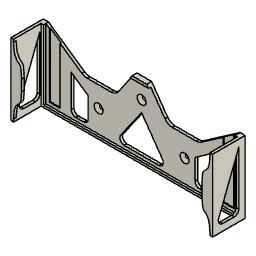
ThinkPad_Dock_Mount_v1 (Autodesk Fusion 360 design; units mm, degrees)
Autodesk Fusion 360 part; units mm, degrees
sketch "Sketch2" plane through (0, 0, 0) normal (0, 0, 1) x (1, 0, 0)
  line L0 (-139.5, 128) -> (87, 128)
  line L1 (87, 128) -> (87, 91.5)
  line L2 (87, 91.5) -> (-139.5, 91.5)
  line L3 (-139.5, 91.5) -> (-139.5, 128)
  line L4 (-136.5, 125) -> (84, 125)
  line L5 (84, 125) -> (84, 94.5)
  line L6 (84, 94.5) -> (-136.5, 94.5)
  line L7 (-136.5, 94.5) -> (-136.5, 125)
  dimension "d3" = 3
  dimension "d4" = 3
  dimension "d5" = 3
  dimension "d6" = 3
  dimension "d7" = 220.5
  dimension "d8" = 30.5
  constraint horizontal L0
  constraint vertical L1
  constraint horizontal L2
  constraint vertical L3
  constraint horizontal L4
  constraint vertical L5
  constraint horizontal L6
  constraint vertical L7
  measures "d3" distance of L0 L4
  measures "d4" distance of L1 L5
  measures "d5" distance of L3 L7
  measures "d6" distance of L2 L6
  measures "d7" distance of L5 L7
  measures "d8" distance of L4 L6
extrude "Extrude1" add sketch "Sketch2" along normal blind 80.5 makes body 1
sketch "Sketch3" plane through (0, 0, 0) normal (0, 0, -1) x (1, 0, 0)
  line L0 (-136.5, -94.5) -> (84, -94.5)
  line L1 (84, -94.5) -> (84, -125)
  line L2 (84, -125) -> (-136.5, -125)
  line L3 (-136.5, -125) -> (-136.5, -94.5)
  line L4 (87, -91.5) -> (-139.5, -91.5)
  line L5 (-139.5, -91.5) -> (-139.5, -128)
  line L6 (-139.5, -128) -> (87, -128)
  line L7 (87, -128) -> (87, -91.5)
  line L8 (-136.5, -125) -> (-133.75, -125)
  line L9 (-133.75, -125) -> (-133.75, -122.5)
  line L10 (-133.75, -122.5) -> (-136.5, -122.5)
  line L11 (-136.5, -122.5) -> (-136.5, -125)
  line L12 (84, -125) -> (81.25, -125)
  line L13 (81.25, -125) -> (81.25, -122.5)
  line L14 (81.25, -122.5) -> (84, -122.5)
  line L15 (84, -122.5) -> (84, -125)
  dimension "d11" = 2.5
  dimension "d12" = 2.75
  dimension "d13" = 2.5
  dimension "d14" = 2.75
  constraint horizontal L8
  constraint vertical L9
  constraint horizontal L10
  constraint vertical L11
  constraint coincident L2.end L3.start
  constraint horizontal L12
  constraint vertical L13
  constraint horizontal L14
  constraint vertical L15
  constraint coincident L1.end L2.start
  measures "d11" distance of L8 L10
  measures "d12" distance of L9 L11
  measures "d13" distance of L12 L14
  measures "d14" distance of L13 L15
extrude "Extrude2" add sketch "Sketch3" against normal blind 80.5 separate body contours L2 L3 L8 L9 L10 L11 | L1 L2 L12 L13 L14 L15 makes body 2 at (-134.6667, 122.5, 53.6667) makes body 3 at (83.0833, 125, 53.6667)
sketch "Sketch4" plane through (-133.75, 0, 0) normal (1, 0, 0) x (0, 1, 0)
  line L0 (122.5, 0) -> (125, 0)
  line L1 (125, 0) -> (125, 80.5)
  line L2 (125, 80.5) -> (122.5, 80.5)
  line L3 (122.5, 80.5) -> (122.5, 0)
  line L4 (122.5, 0) -> (125, 0)
  line L5 (125, 0) -> (125, 2.5)
  line L6 (125, 2.5) -> (122.5, 2.5)
  line L7 (122.5, 2.5) -> (122.5, 0)
  dimension "d17" = 2.5
  constraint horizontal L4
  constraint vertical L5
  constraint horizontal L6
  constraint vertical L7
  constraint coincident L1 L5.end
  constraint coincident L0.start L3.end
  measures "d17" distance of L4 L6
extrude "Extrude3" add sketch "Sketch4" along normal up to surface (215 mm away) contours L0 L1 L3 L4 L5 L6 L7 bodies 1 2 3
sketch "Sketch34" plane through (0, 91.5, 0) normal (0, -1, 0) x (1, 0, 0)
  line L0 (-139.5, 0) -> (87, 0)
  line L1 (-139.5, 80.5) -> (-139.5, 0)
  line L2 (-136.5, 2.753) -> (-136.5, 0)
  line L3 (-139.5, 40.25) -> (-127.5, 40.25)
  line L4 (-26.25, 0) -> (-26.25, 10)
  line L5 (-127.5, 40.25) -> (-127.5, 34.253)
  spline S0 degree 5 poles (-127.5, 34.253) (-127.5, 33.9218) (-127.5144, 33.2317) (-127.5794, 32.1133) (-127.7268, 30.4836) (-127.9198, 28.3513) (-128.0379, 26.2907) (-128.1709, 24.3948) (-128.4617, 22.7323) (-129.6807, 21.0236) (-131.358, 19.6123) (-132.5708, 18.9131) (-132.5285, 19.155) (-132.375, 19.0496) (-133.1587, 17.6828) (-134.3735, 15.6105) (-135.3998, 13.5294) (-135.6827, 12.0317) (-135.798, 10.5363) (-135.9647, 8.8274) (-136.2123, 6.8844) (-136.4008, 5.2251) (-136.482, 3.9805) (-136.5, 3.1606) (-136.5, 2.753) knots 0 0 0 0 0 0 0.05 0.1 0.15 0.2 0.25 0.3 0.35 0.4 0.45 0.5 0.55 0.6 0.65 0.7 0.75 0.8 0.85 0.9 0.95 1 1 1 1 1 1
  line L6 (-127.5, 37.2515) -> (-127.5, 31.2546)
  line L7 (-136.5, 6.6399) -> (-136.5, -1.1338)
  line L8 (-127.3272, 26.6249) -> (-129.6728, 19.7501)
  line L9 (-132.4893, 19.089) -> (-132.5107, 19.0556)
  line L10 (-134.7118, 16.064) -> (-136.2882, 9.4421)
  line L11 (-136.5, 77.747) -> (-136.5, 80.5)
  spline S1 degree 5 poles (-127.5, 46.247) (-127.5, 46.5782) (-127.5144, 47.2683) (-127.5794, 48.3867) (-127.7268, 50.0164) (-127.9198, 52.1487) (-128.0379, 54.2093) (-128.1709, 56.1052) (-128.4617, 57.7677) (-129.6807, 59.4764) (-131.358, 60.8877) (-132.5708, 61.5869) (-132.5285, 61.345) (-132.375, 61.4504) (-133.1587, 62.8172) (-134.3735, 64.8895) (-135.3998, 66.9706) (-135.6827, 68.4683) (-135.798, 69.9637) (-135.9647, 71.6726) (-136.2123, 73.6156) (-136.4008, 75.2749) (-136.482, 76.5195) (-136.5, 77.3394) (-136.5, 77.747) knots 0 0 0 0 0 0 0.05 0.1 0.15 0.2 0.25 0.3 0.35 0.4 0.45 0.5 0.55 0.6 0.65 0.7 0.75 0.8 0.85 0.9 0.95 1 1 1 1 1 1
  line L12 (-127.5, 43.2485) -> (-127.5, 49.2454)
  line L13 (-127.3272, 53.8751) -> (-129.6728, 60.7499)
  line L14 (-132.4893, 61.411) -> (-132.5107, 61.4444)
  line L15 (-134.7118, 64.436) -> (-136.2882, 71.0579)
  line L16 (-136.5, 73.8601) -> (-136.5, 81.6338)
  line L17 (-127.5, 40.25) -> (-127.5, 46.247)
  line L18 (84, 2.753) -> (84, 0)
  spline S2 degree 5 poles (75, 34.253) (75, 33.9218) (75.0144, 33.2317) (75.0794, 32.1133) (75.2268, 30.4836) (75.4198, 28.3513) (75.5379, 26.2907) (75.6709, 24.3948) (75.9617, 22.7323) (77.1807, 21.0236) (78.858, 19.6123) (80.0708, 18.9131) (80.0285, 19.155) (79.875, 19.0496) (80.6587, 17.6828) (81.8735, 15.6105) (82.8998, 13.5294) (83.1827, 12.0317) (83.298, 10.5363) (83.4647, 8.8274) (83.7123, 6.8844) (83.9008, 5.2251) (83.982, 3.9805) (84, 3.1606) (84, 2.753) knots 0 0 0 0 0 0 0.05 0.1 0.15 0.2 0.25 0.3 0.35 0.4 0.45 0.5 0.55 0.6 0.65 0.7 0.75 0.8 0.85 0.9 0.95 1 1 1 1 1 1
  line L19 (75, 37.2515) -> (75, 31.2546)
  line L20 (74.8272, 26.6249) -> (77.1728, 19.7501)
  line L21 (79.9893, 19.089) -> (80.0107, 19.0556)
  line L22 (82.2118, 16.064) -> (83.7882, 9.4421)
  line L23 (84, 6.6399) -> (84, -1.1338)
  line L24 (75, 40.25) -> (75, 34.253)
  line L25 (75, 40.25) -> (75, 46.247)
  spline S3 degree 5 poles (75, 46.247) (75, 46.5782) (75.0144, 47.2683) (75.0794, 48.3867) (75.2268, 50.0164) (75.4198, 52.1487) (75.5379, 54.2093) (75.6709, 56.1052) (75.9617, 57.7677) (77.1807, 59.4764) (78.858, 60.8877) (80.0708, 61.5869) (80.0285, 61.345) (79.875, 61.4504) (80.6587, 62.8172) (81.8735, 64.8895) (82.8998, 66.9706) (83.1827, 68.4683) (83.298, 69.9637) (83.4647, 71.6726) (83.7123, 73.6156) (83.9008, 75.2749) (83.982, 76.5195) (84, 77.3394) (84, 77.747) knots 0 0 0 0 0 0 0.05 0.1 0.15 0.2 0.25 0.3 0.35 0.4 0.45 0.5 0.55 0.6 0.65 0.7 0.75 0.8 0.85 0.9 0.95 1 1 1 1 1 1
  line L26 (75, 43.2485) -> (75, 49.2454)
  line L27 (74.8272, 53.8751) -> (77.1728, 60.7499)
  line L28 (79.9893, 61.411) -> (80.0107, 61.4444)
  line L29 (82.2118, 64.436) -> (83.7882, 71.0579)
  line L30 (84, 73.8601) -> (84, 81.6338)
  line L31 (84, 77.747) -> (84, 80.5)
  line L32 (-139.5, 80.5) -> (87, 80.5)
  point P0 (-127.5, 34.253)
  point P1 (-128.5, 23.1875)
  point P2 (-132.5, 19.0723)
  point P3 (-135.5, 12.753)
  point P4 (-136.5, 2.753)
  point P5 (-128.5, 23.1875)
  point P6 (-132.5, 19.0723)
  point P7 (-135.5, 12.753)
  point P8 (-128.5, 57.3125)
  point P9 (-132.5, 61.4277)
  point P10 (-135.5, 67.747)
  point P11 (76, 23.1875)
  point P12 (80, 19.0723)
  point P13 (83, 12.753)
  point P14 (76, 57.3125)
  point P15 (80, 61.4277)
  point P16 (83, 67.747)
  dimension "d201" = 3
  dimension "d255" = 12
  dimension "d257" = 11
  dimension "d259" = 7
  dimension "d261" = 4
  dimension "d263" = 3
  dimension "d265" = 3
  dimension "d266" = 18.839
  dimension "d267" = 32.677
  dimension "d268" = 13.391
  dimension "d274" = 41.3838
  constraint coincident L0 L2.end
  constraint midpoint L1 L3.start
  constraint perpendicular L1 L3
  constraint midpoint L0 L4.start
  constraint perpendicular L0 L4
  constraint coincident P0 L5.end
  constraint perpendicular L3 L5
  constraint coincident P5 P1
  constraint coincident P6 P2
  constraint coincident P7 P3
  constraint midpoint P0 L6
  constraint midpoint L5 L6.start
  constraint midpoint L2.start L7
  constraint midpoint P5 L8
  constraint midpoint P6 L9
  constraint midpoint P7 L10
  constraint parallel L1 L7
  constraint symmetric L2.start L3 L11.start
  constraint symmetric L2.end L3 L11.end
  constraint symmetric L5.start L3 L17.start
  constraint symmetric L3 P0 S1.start
  constraint symmetric L3 P5 P8
  constraint symmetric L3 P6 P9
  constraint symmetric L3 P7 P10
  constraint symmetric L3 L6.start L12.start
  constraint symmetric L3 L6.end L12.end
  constraint symmetric L3 L7.start L16.start
  constraint symmetric L3 L7.end L16.end
  constraint symmetric L3 L8.start L13.start
  constraint symmetric L3 L8.end L13.end
  constraint symmetric L3 L9.start L14.start
  constraint symmetric L3 L9.end L14.end
  constraint symmetric L3 L10.start L15.start
  constraint symmetric L3 L10.end L15.end
  constraint symmetric L2.start L4 L18.start
  constraint symmetric L2.end L4 L18.end
  constraint symmetric L3.end L4 L24.start
  constraint symmetric L4 P0 S2.start
  constraint symmetric L4 P5 P11
  constraint symmetric L4 P6 P12
  constraint symmetric L4 P7 P13
  constraint symmetric L4 L6.start L19.start
  constraint symmetric L4 L6.end L19.end
  constraint symmetric L4 L7.start L23.start
  constraint symmetric L4 L7.end L23.end
  constraint symmetric L4 L8.start L20.start
  constraint symmetric L4 L8.end L20.end
  constraint symmetric L4 L9.start L21.start
  constraint symmetric L4 L9.end L21.end
  constraint symmetric L4 L10.start L22.start
  constraint symmetric L4 L10.end L22.end
  constraint symmetric L4 L11.start S3.end
  constraint symmetric L4 L11.end L31.end
  constraint symmetric L4 S1.start L25.end
  constraint symmetric L4 P8 P14
  constraint symmetric L4 P9 P15
  constraint symmetric L4 P10 P16
  constraint symmetric L4 L12.start L26.start
  constraint symmetric L4 L12.end L26.end
  constraint symmetric L4 L13.start L27.start
  constraint symmetric L4 L13.end L27.end
  constraint symmetric L4 L14.start L28.start
  constraint symmetric L4 L14.end L28.end
  constraint symmetric L4 L15.start L29.start
  constraint symmetric L4 L15.end L29.end
  constraint symmetric L4 L16.start L30.start
  constraint symmetric L4 L16.end L30.end
  constraint symmetric L4 L3.end L24.start
  measures "d201" distance of L1 L2.end
  measures "d255" distance of L1 P0
  measures "d257" distance of L1 P5
  measures "d259" distance of L1 P6
  measures "d261" distance of L1 P7
  measures "d263" distance of L1 P4
  measures "d265" distance of L1 L7.end
  measures "d266" angle of L1 L8
  measures "d267" angle of L1 L9
  measures "d268" angle of L1 L10
  measures "d274" distance of L3 L7.end
extrude "Extrude20" cut sketch "Sketch34" against normal blind 3 contours L0 L2 L5 S0 L6 L7 L11 S1 L12 L16 L17 L18 S2 L19 L23 L24 L25 S3 L26 L30 L31 L32 bodies 1
sketch "Sketch6" plane through (0, 125, 0) normal (0, -1, 0) x (1, 0, 0)
  line L0 (-133.75, 2.5) -> (81.25, 2.5)
  line L1 (81.25, 2.5) -> (81.25, 80.5)
  line L2 (81.25, 80.5) -> (-133.75, 80.5)
  line L3 (-133.75, 80.5) -> (-133.75, 2.5)
  line L4 (-133.75, 80.5) -> (-93.2117, 52.2917)
  arc A0 (-93.2117, 52.2917) -> (-87.5, 50.5) centre (-87.5, 60.5) ccw
  line L5 (-52.4841, 54.771) -> (-34.5, 80.5)
  line L6 (-87.5, 50.5) -> (-60.6803, 50.5)
  arc A1 (-60.6803, 50.5) -> (-52.4841, 54.771) centre (-60.6803, 60.5) ccw
  line L7 (-26.25, 80.5) -> (-26.25, 2.5)
  line L8 (-0.0159, 54.771) -> (-18, 80.5)
  arc A2 (-0.0159, 54.771) -> (8.1803, 50.5) centre (8.1803, 60.5) ccw
  line L9 (35, 50.5) -> (8.1803, 50.5)
  arc A3 (35, 50.5) -> (40.7117, 52.2917) centre (35, 60.5) ccw
  line L10 (81.25, 80.5) -> (40.7117, 52.2917)
  point P0 (-55.4694, 50.5)
  dimension "d81" = 10
  dimension "d86" = 10
  dimension "d143" = 8.25
  dimension "d144" = 34.4303
  dimension "d156" = 61.25
  dimension "d236" = 30
  constraint perpendicular L3 L6
  constraint tangent L4 A0
  constraint tangent A0 L6
  constraint coincident L2 L5.end
  constraint coincident P0 L5
  constraint coincident P0 L6
  constraint tangent L5 A1
  constraint tangent L6 A1
  constraint midpoint L2 L7.start
  constraint midpoint L0 L7.end
  constraint coincident L2.end L3.start
  constraint symmetric L4.end L7 A3.end
  constraint symmetric A0.end L7 L9.start
  constraint symmetric A0 L7 A3
  constraint symmetric L5.end L7 L8.end
  constraint symmetric L5.start L7 L8.start
  constraint symmetric L6.end L7 A2.end
  constraint symmetric A1 L7 A2
  constraint symmetric L7 L2.end L1.end
  measures "d81" radius of A0
  measures "d86" radius of A1
  measures "d143" distance of L5.end L7.start
  measures "d144" horizontal distance of A1.centre L7.start
  measures "d156" horizontal distance of A0.centre L7.start
  measures "d236" distance of L2 L6
sketch "Sketch29" plane through (0, 125, 0) normal (0, -1, 0) x (1, 0, 0)
  line L0 (-133.75, 2.5) -> (81.25, 2.5)
  line L1 (81.25, 2.5) -> (81.25, 80.5)
  line L2 (81.25, 80.5) -> (-133.75, 80.5)
  line L3 (-133.75, 80.5) -> (-133.75, 2.5)
  line L4 (-26.25, 2.5) -> (-26.25, 60)
  point P0 (-26.25, 60)
  point P1 (-74.5, 27.5)
  point P2 (22, 27.5)
  dimension "d181" = 57.5
  dimension "d182" = 48.25
  dimension "d183" = 25
  constraint midpoint L0 L4.start
  constraint perpendicular L0 L4
  constraint coincident P0 L4.end
  constraint symmetric L4 P1 P2
  measures "d181" distance of L4.start P0
  measures "d182" distance of L4 P1
  measures "d183" distance of L0 P1
extrude "Extrude5" cut sketch "Sketch6" against normal blind 3 contours L2 L4 A0 L5 L6 A1 | L2 L8 A2 L9 A3 L10 bodies 1
sketch "Sketch21" plane through (0, 125, 0) normal (0, -1, 0) x (1, 0, 0)
  line L0 (-93.2117, 52.2917) -> (-133.75, 80.5)
  line L1 (-133.75, 80.5) -> (-133.75, 2.5)
  line L2 (-133.75, 2.5) -> (81.25, 2.5)
  line L3 (81.25, 2.5) -> (81.25, 80.5)
  line L4 (-18, 80.5) -> (-34.5, 80.5)
  line L5 (-34.5, 80.5) -> (-52.4841, 54.771)
  arc A0 (-60.6803, 50.5) -> (-52.4841, 54.771) centre (-60.6803, 60.5) ccw
  line L6 (-60.6803, 50.5) -> (-87.5, 50.5)
  arc A1 (-93.2117, 52.2917) -> (-87.5, 50.5) centre (-87.5, 60.5) ccw
  line L7 (-129.75, 83.0225) -> (-117.75, 83.0225)
  line L8 (-117.75, 83.0225) -> (-117.75, 6)
  line L9 (-117.75, 6) -> (-129.75, 6)
  line L10 (-129.75, 6) -> (-129.75, 83.0225)
  line L11 (-136.5, 0) -> (84, 0)
  line L12 (-26.25, 2.5) -> (-26.25, 27.8547)
  line L13 (77.25, 6) -> (77.25, 83.0225)
  line L14 (77.25, 83.0225) -> (65.25, 83.0225)
  line L15 (65.25, 83.0225) -> (65.25, 6)
  line L16 (65.25, 6) -> (77.25, 6)
  line L17 (81.25, 80.5) -> (40.7117, 52.2917)
  arc A2 (35, 50.5) -> (40.7117, 52.2917) centre (35, 60.5) ccw
  line L18 (35, 50.5) -> (8.1803, 50.5)
  arc A3 (-0.0159, 54.771) -> (8.1803, 50.5) centre (8.1803, 60.5) ccw
  line L19 (-0.0159, 54.771) -> (-18, 80.5)
  dimension "d163" = 12
  dimension "d165" = 6
  dimension "d173" = 103.5
  constraint horizontal L7
  constraint vertical L8
  constraint horizontal L9
  constraint vertical L10
  constraint midpoint L2 L12.start
  constraint perpendicular L2 L12
  constraint symmetric L7.start L12 L13.end
  constraint symmetric L7.end L12 L14.end
  constraint symmetric L8.end L12 L15.end
  constraint symmetric L9.end L12 L13.start
  measures "d163" distance of L7.start L7.end
  measures "d165" distance of L9 L11
  measures "d173" distance of L10 L12
extrude "Extrude16" cut sketch "Sketch21" against normal blind 1 contours L0 L8 L9 L10 | L13 L15 L16 L17 bodies 1
sketch "Sketch25" plane through (0, 125, 0) normal (0, -1, 0) x (1, 0, 0)
  line L0 (-129.75, 6) -> (-129.75, 77.7166)
  line L1 (-129.75, 77.7166) -> (-133.75, 80.5)
  line L2 (-133.75, 80.5) -> (-133.75, 2.5)
  line L3 (-133.75, 2.5) -> (81.25, 2.5)
  line L4 (81.25, 2.5) -> (81.25, 80.5)
  line L5 (81.25, 80.5) -> (77.25, 77.7166)
  line L6 (77.25, 77.7166) -> (77.25, 6)
  line L7 (77.25, 6) -> (65.25, 6)
  line L8 (65.25, 6) -> (65.25, 69.3665)
  arc A0 (35, 50.5) -> (40.7117, 52.2917) centre (35, 60.5) ccw
  line L9 (35, 50.5) -> (8.1803, 50.5)
  arc A1 (-0.0159, 54.771) -> (8.1803, 50.5) centre (8.1803, 60.5) ccw
  line L10 (-0.0159, 54.771) -> (-18, 80.5)
  line L11 (-18, 80.5) -> (-34.5, 80.5)
  line L12 (-34.5, 80.5) -> (-52.4841, 54.771)
  arc A2 (-60.6803, 50.5) -> (-52.4841, 54.771) centre (-60.6803, 60.5) ccw
  line L13 (-60.6803, 50.5) -> (-87.5, 50.5)
  arc A3 (-93.2117, 52.2917) -> (-87.5, 50.5) centre (-87.5, 60.5) ccw
  line L14 (-117.75, 69.3665) -> (-117.75, 6)
  line L15 (-117.75, 6) -> (-129.75, 6)
  line L16 (-36.5969, 77.5) -> (-15.9031, 77.5)
  line L17 (65.25, 69.3665) -> (40.7117, 52.2917)
  line L18 (-93.2117, 52.2917) -> (-117.75, 69.3665)
  dimension "d177" = 3
  constraint horizontal L16
  constraint coincident L10 L16.end
  constraint coincident L12 L16.start
  measures "d177" distance of L11 L16
extrude "Extrude18" add sketch "Sketch25" along normal blind 2.5 contours L10 L11 L12 L16 bodies 1
hole "Hole1" at (-74.5, 125, 27.5) at (-26.25, 125, 60) at (22, 125, 27.5) direction (0, 1, 0) diameter 3.5 depth 8 tip angle 180 countersink diameter 10 countersink angle 90 bodies 1
sketch "Sketch35" plane through (0, 125, 0) normal (0, -1, 0) x (1, 0, 0)
  circle A0 centre (-26.25, 60) radius 5
  circle A1 centre (-74.5, 27.5) radius 5
  circle A2 centre (22, 27.5) radius 5
  line L0 (-15.9031, 77.5) -> (-36.5969, 77.5)
  line L1 (-36.5969, 77.5) -> (-52.4841, 54.771)
  arc A3 (-60.6803, 50.5) -> (-52.4841, 54.771) centre (-60.6803, 60.5) ccw
  line L2 (-60.6803, 50.5) -> (-87.5, 50.5)
  arc A4 (-93.2117, 52.2917) -> (-87.5, 50.5) centre (-87.5, 60.5) ccw
  line L3 (-117.75, 69.3665) -> (-117.75, 6)
  line L4 (-117.75, 6) -> (-129.75, 6)
  line L5 (-129.75, 6) -> (-129.75, 77.7166)
  line L6 (-93.2117, 52.2917) -> (-117.75, 69.3665)
  line L7 (-133.75, 80.5) -> (-133.75, 2.5)
  line L8 (-133.75, 2.5) -> (81.25, 2.5)
  line L9 (81.25, 2.5) -> (81.25, 80.5)
  line L10 (81.25, 80.5) -> (77.25, 77.7166)
  line L11 (77.25, 77.7166) -> (77.25, 6)
  line L12 (77.25, 6) -> (65.25, 6)
  line L13 (65.25, 6) -> (65.25, 69.3665)
  arc A5 (35, 50.5) -> (40.7117, 52.2917) centre (35, 60.5) ccw
  line L14 (35, 50.5) -> (8.1803, 50.5)
  arc A6 (-0.0159, 54.771) -> (8.1803, 50.5) centre (8.1803, 60.5) ccw
  line L15 (-0.0159, 54.771) -> (-15.9031, 77.5)
  line L16 (-45.6625, 6) -> (-6.8375, 6)
  line L17 (-2.7394, 13.8645) -> (-26.25, 47.5)
  line L18 (-26.25, 47.5) -> (-49.7606, 13.8645)
  arc A7 (-49.7606, 13.8645) -> (-45.6625, 6) centre (-45.6625, 11) ccw
  arc A8 (-6.8375, 6) -> (-2.7394, 13.8645) centre (-6.8375, 11) ccw
  line L19 (65.25, 69.3665) -> (40.7117, 52.2917)
  line L20 (-129.75, 77.7166) -> (-133.75, 80.5)
  dimension "d217" = 3.5
  dimension "d218" = 41.5
  dimension "d219" = 48.25
  dimension "d220" = 5
  constraint horizontal L16
  constraint tangent L16 A7
  constraint tangent L18 A7
  constraint tangent L16 A8
  constraint tangent L17 A8
  constraint equal A7 A8
  constraint parallel L15 L17
  constraint parallel L1 L18
  measures "d217" distance of L8 L16
  measures "d218" distance of L16 L17.end
  measures "d219" horizontal distance of A2.centre L17.end
  measures "d220" radius of A7
extrude "Extrude21" cut sketch "Sketch35" against normal blind 10 contours L16 L17 L18 A7 A8 bodies 1
sketch "Sketch37" plane through (0, 125, 0) normal (0, -1, 0) x (1, 0, 0)
  line L0 (-26.25, 47.5) -> (-2.7394, 13.8645)
  arc A0 (-6.8375, 6) -> (-2.7394, 13.8645) centre (-6.8375, 11) ccw
  line L1 (-6.8375, 6) -> (-45.6625, 6)
  arc A1 (-49.7606, 13.8645) -> (-45.6625, 6) centre (-45.6625, 11) ccw
  line L2 (-49.7606, 13.8645) -> (-26.25, 47.5)
  circle A2 centre (-26.25, 60) radius 5
  circle A3 centre (-74.5, 27.5) radius 5
  circle A4 centre (22, 27.5) radius 5
  line L3 (-15.9031, 77.5) -> (-36.5969, 77.5)
  line L4 (-36.5969, 77.5) -> (-52.4841, 54.771)
  arc A5 (-60.6803, 50.5) -> (-52.4841, 54.771) centre (-60.6803, 60.5) ccw
  line L5 (-60.6803, 50.5) -> (-87.5, 50.5)
  arc A6 (-93.2117, 52.2917) -> (-87.5, 50.5) centre (-87.5, 60.5) ccw
  line L6 (-117.75, 69.3665) -> (-117.75, 6)
  line L7 (-117.75, 6) -> (-129.75, 6)
  line L8 (-129.75, 6) -> (-129.75, 77.7166)
  line L9 (-93.2117, 52.2917) -> (-117.75, 69.3665)
  line L10 (-133.75, 80.5) -> (-133.75, 2.5)
  line L11 (-133.75, 2.5) -> (81.25, 2.5)
  line L12 (81.25, 2.5) -> (81.25, 80.5)
  line L13 (81.25, 80.5) -> (77.25, 77.7166)
  line L14 (77.25, 77.7166) -> (77.25, 6)
  line L15 (77.25, 6) -> (65.25, 6)
  line L16 (65.25, 6) -> (65.25, 69.3665)
  arc A7 (35, 50.5) -> (40.7117, 52.2917) centre (35, 60.5) ccw
  line L17 (35, 50.5) -> (8.1803, 50.5)
  arc A8 (-0.0159, 54.771) -> (8.1803, 50.5) centre (8.1803, 60.5) ccw
  line L18 (-0.0159, 54.771) -> (-15.9031, 77.5)
  line L19 (-86.25, 11) -> (-86.25, 34.0464)
  line L20 (-86.25, 34.0464) -> (-105.25, 47.2674)
  line L21 (-105.25, 47.2674) -> (-105.25, 11)
  line L22 (-100.25, 6) -> (-91.25, 6)
  arc A9 (-105.25, 11) -> (-100.25, 6) centre (-100.25, 11) ccw
  arc A10 (-91.25, 6) -> (-86.25, 11) centre (-91.25, 11) ccw
  line L23 (-26.25, 2.5) -> (-26.25, 51)
  line L24 (33.75, 34.0464) -> (52.75, 47.2674)
  line L25 (52.75, 47.2674) -> (52.75, 11)
  line L26 (47.75, 6) -> (38.75, 6)
  arc A11 (47.75, 6) -> (52.75, 11) centre (47.75, 11) ccw
  arc A12 (33.75, 11) -> (38.75, 6) centre (38.75, 11) ccw
  line L27 (33.75, 11) -> (33.75, 34.0464)
  line L28 (65.25, 69.3665) -> (40.7117, 52.2917)
  line L29 (-129.75, 77.7166) -> (-133.75, 80.5)
  dimension "d223" = 11.75
  dimension "d224" = 3.5
  dimension "d225" = 19
  dimension "d226" = 5
  dimension "d275" = 11
  constraint vertical L19
  constraint parallel L19 L21
  constraint perpendicular L19 L22
  constraint tangent L21 A9
  constraint tangent L22 A9
  constraint tangent L19 A10
  constraint tangent L22 A10
  constraint equal A9 A10
  constraint midpoint L11 L23.start
  constraint perpendicular L11 L23
  constraint symmetric L19.end L23 L24.start
  constraint symmetric L20.end L23 L24.end
  constraint symmetric L21.end L23 L25.end
  constraint symmetric L22.start L23 L26.start
  constraint symmetric A9 L23 A11
  constraint symmetric L19.start L23 A12.start
  constraint symmetric L22.end L23 L26.end
  constraint symmetric A10 L23 A12
  constraint parallel L9 L20
  measures "d223" distance of A3.centre L19
  measures "d224" distance of L11 L22
  measures "d225" distance of L19 L21
  measures "d226" radius of A9
  measures "d275" distance of L9 L20.end
extrude "Extrude22" cut sketch "Sketch37" against normal blind 10 contours L19 L20 L21 L22 A9 A10 | L24 L25 L26 A11 A12 L27 bodies 1
sketch "Sketch38" plane through (-139.5, 0, 0) normal (-1, 0, 0) x (0, -1, 0)
  line L0 (-128, 0) -> (-91.5, 0)
  line L1 (-91.5, 0) -> (-91.5, 80.5)
  line L2 (-91.5, 80.5) -> (-128, 80.5)
  line L3 (-128, 80.5) -> (-128, 0)
  line L4 (-116, 7.5) -> (-102.8121, 7.5)
  line L5 (-98.1528, 14.3139) -> (-121, 73)
  line L6 (-121, 73) -> (-121, 12.5)
  arc A0 (-121, 12.5) -> (-116, 7.5) centre (-116, 12.5) ccw
  arc A1 (-102.8121, 7.5) -> (-98.1528, 14.3139) centre (-102.8121, 12.5) ccw
  point P0 (-95.5, 7.5)
  dimension "d230" = 7
  dimension "d231" = 4
  dimension "d232" = 7.5
  dimension "d233" = 7.5
  dimension "d234" = 5
  constraint horizontal L4
  constraint perpendicular L4 L6
  constraint tangent L4 A0
  constraint tangent L6 A0
  constraint coincident P0 L4
  constraint coincident P0 L5
  constraint tangent L4 A1
  constraint tangent L5 A1
  constraint equal A0 A1
  measures "d230" distance of L3 L6
  measures "d231" distance of L1 P0
  measures "d232" distance of L0 L4
  measures "d233" distance of L2 L5.end
  measures "d234" radius of A0
extrude "Extrude23" cut sketch "Sketch38" against normal through all contours L4 L5 L6 A0 A1 bodies 1
equation "d7 = DOCK_WIDTH + 0.5 mm"
equation "d8 = DOCK_HEIGHT + 0.5 mm"
equation "d9 = DOCK_DEPTH + 0.5 mm"
equation "d15 = -DOCK_DEPTH - 0.5 mm"
equation "DOCK_WIDTH = 220 mm"
equation "DOCK_HEIGHT = 30 mm"
equation "d173 = DOCK_WIDTH / 2 - 6.5 mm"
equation "DOCK_DEPTH = 80 mm"
equation "d181 = 60 mm - 2.5 mm"
